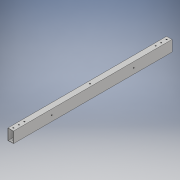
# Autodesk Inventor part: 1x1 29in
Saved by Autodesk Inventor 2018 (Build 220112000, 112)
## iProperties
Created: 2019-01-13
Part Number: 1x1 29in
Material: Generic
Document SubType Name: Modeling
Designer: s-2512711
Density: 1 g/cm^3
Appearance: Default
Author: s-2512711
Autodesk Inventor part; units mm, degrees
ref_plane "YZ Plane" through (0, 0, 0) normal (1, 0, 0) x (0, 1, 0)
ref_plane "XZ Plane" through (0, 0, 0) normal (0, 1, 0) x (-1, 0, 0)
ref_plane "XY Plane" through (0, 0, 0) normal (0, 0, 1) x (1, 0, 0)
sketch "Sketch1" plane through (0, 0, 0) normal (0, 0, 1) x (1, 0, 0)
  line L0 (0, 0) -> (25.4, 0)
  line L1 (25.4, 0) -> (25.4, 50.8)
  line L2 (25.4, 50.8) -> (0, 50.8)
  line L3 (0, 50.8) -> (0, 0)
  line L4 (1.5875, 49.2125) -> (23.8125, 49.2125)
  line L5 (23.8125, 49.2125) -> (23.8125, 1.5875)
  line L6 (23.8125, 1.5875) -> (1.5875, 1.5875)
  line L7 (1.5875, 1.5875) -> (1.5875, 49.2125)
  dimension "d0" = 25.4
  dimension "d1" = 50.8
  dimension "d2" = 1.5875
  constraints: 16 end point, 4 parallel, 2 perpendicular, 1 horizontal, 3 other
  measures "d0" distance of L2.end L1.end
  measures "d1" distance of L1.end L0.end
  measures "d2" distance between parallel lines of L2 L4
extrude "Extrusion1" add sketch "Sketch1" along normal blind 736.6
sketch "Sketch2" plane through (25.4, 0, 0) normal (1, 0, 0) x (0, 0, -1)
  line L0 (0, 49.2125) -> (0, 1.5875) construction
  line L1 (0, 25.4) -> (-177.8, 25.4) construction
  line L2 (-736.6, 50.8) -> (-736.6, 0) construction
  line L3 (-736.6, 25.4) -> (-558.8, 25.4) construction
  circle A0 centre (-558.8, 25.4) radius 2.5797
  circle A1 centre (-177.8, 25.4) radius 2.5797
  point P0 (0, 0)
  dimension "d5" = 177.8
  dimension "d6" = 177.8
  dimension "d7" = 5.1594
  constraints: 4 end point, 2 centre point, 2 coincident, 2 horizontal, 2 midpoint
  measures "d5" distance of L1.start L1.end
  measures "d6" distance of L3.start L3.end
  measures "d7" diameter of A0
extrude "Extrusion2" cut sketch "Sketch2" against normal blind 25.4
sketch "Sketch3" plane through (0, 50.8, 0) normal (0, 1, 0) x (1, 0, 0)
  line L0 (0, 0) -> (0, -736.6) construction
  line L1 (0, -368.3) -> (25.4, -368.3) construction
  line L2 (0, -368.3) -> (25.4, -368.3) construction
  circle A0 centre (12.7, -368.3) radius 2.5797
  dimension "d10" = 25.4
  dimension "d11" = 0
  dimension "d12" = 5.1594
  constraints: 4 end point, 2 midpoint, 1 centre point, 1 collinear, 1 horizontal, 1 perpendicular
  measures "d10" distance of L1.start L1.end
  measures "d11" distance between parallel lines of L1 L2
  measures "d12" diameter of A0
extrude "Extrusion3" cut sketch "Sketch3" against normal blind 25.4
sketch "Sketch4" plane through (0, 50.8, 0) normal (0, 1, 0) x (1, 0, 0)
  line L0 (1.5875, 0) -> (23.8125, 0) construction
  line L1 (12.7, 0) -> (12.7, -12.7) construction
  line L2 (12.7, -12.7) -> (12.7, -38.1) construction
  line L3 (12.7, -38.1) -> (12.7, -63.5) construction
  line L4 (0, 0) -> (0, -736.6) construction
  line L5 (0, -368.3) -> (25.4, -368.3) construction
  line L6 (25.4, 0) -> (25.4, -736.6) construction
  circle A0 centre (12.7, -12.7) radius 2.5797
  circle A1 centre (12.7, -38.1) radius 2.5797
  circle A2 centre (12.7, -63.5) radius 2.5797
  circle A3 centre (12.7, -723.9) radius 2.5797
  circle A4 centre (12.7, -698.5) radius 2.5797
  circle A5 centre (12.7, -673.1) radius 2.5797
  dimension "d15" = 12.7
  dimension "d16" = 25.4
  dimension "d17" = 25.4
  dimension "d18" = 5.1594
  constraints: 8 end point, 6 centre point, 3 coincident, 3 midpoint, 3 symmetric about line, 2 point on line, 1 vertical, 3 other
  measures "d15" distance of L1.start L1.end
  measures "d16" distance of L1.end L2.end
  measures "d17" distance of L2.end L3.end
  measures "d18" diameter of A0
extrude "Extrusion4" cut sketch "Sketch4" against normal blind 152.4
body "Solid1"
